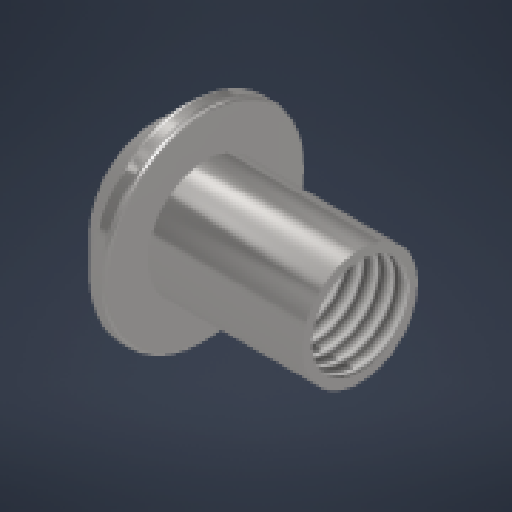
# Autodesk Inventor part: AliM5-8mm
Saved by Autodesk Inventor 2024.3 (Build 283343000, 343)
## iProperties
Created: 2024-06-23
Part Number: AliM5-8mm
Material: 스테인리스스틸
Catalog Web Link: www.cadenas.de
Description: DBB, DBM, DBS, DBSY-Stepped Screws - Low Head Selectable
Vendor: MISUMI
Document SubType Name: Modeling
Designer: ASUS
Manufacturer: MISUMI
Mass: 3.5682 g
Surface Area: 4.58831 cm^2
Volume: 0.446026 cm^3
Density: 8 g/cm^3
Appearance: 반연마
Category: PARTsolutions
Company: MISUMI
Title: DBSY4-5-8
Author: Cadenas PARTsolutions
Comments: Stepped Screws - Low Head Selectable
PSOL_IDENT_0: {$CADENAS_DATA/23d-libs/misumi/metric/27_screws_nuts/dbb.prj},184 {VTYP=3D},{NB=DBSY4-5-8},{LINA=DBS
PSOL_IDENT_1: Y4-5-8},{NN=DBB, DBM, DBS, DBSY},{DATE=29.05.2023 07:54:54},{GEOMDATE=17.01.2022 08:24:34},{VERSION=
PSOL_IDENT_2: },{LINEID=20},{WBVAR=MAT,ST,L,F},{WBNUMERIC=L,F}  {NB=DBSY4-5-8},{LINA=DBSY4-5-8},{KT=DUMMY},{PN=DBS
PSOL_IDENT_3: Y4-5-8},{TYPE=DB},{MAT=SY},{ST=-},{STALG= '-','-'},{M=4},{L=5},{LALG=3,4,5,6,7,8,10},{F=8},{FALG=4,5
PSOL_IDENT_4: ,6,8},{E=2.8},{DHH7=6},{A=10},{B=2.5},{LL=1.2},{HH1=2.5}
NB: DBSY4-5-8
NN: DBB, DBM, DBS, DBSY
NT: Stepped Screws - Low Head Selectable
NBSYN: $PN.
LINA: DBSY4-5-8
CATALOG: Misumi
PN: DBSY4-5-8
TYPE: DB
MAT: 304 Stainless Steel
ST: -
M: 4
L: 5
F: 8
E: 2.8
DHH7: 6
A: 10
B: 2.5
LL: 1.2
HH1: 2.5
SUPPLIER: MISUMI
ARTICLENO: DBSY4-5-8
BOMINFO: DBSY4-5-8
CREATOR: CADENAS GmbH
Autodesk Inventor part; units mm, degrees
ref_plane "YZ Plane" through (0, 0, 0) normal (1, 0, 0) x (0, 1, 0)
ref_plane "XZ Plane" through (0, 0, 0) normal (0, 1, 0) x (-1, 0, 0)
ref_plane "XY Plane" through (0, 0, 0) normal (0, 0, 1) x (1, 0, 0)
sketch "Sketch_1" plane through (0, 0, 0) normal (0, 0, 1) x (1, 0, 0)
  line L0 (8, 0) -> (-7.8, 0)
  line L1 (-7.8, 0) -> (-7.8, 5)
  line L2 (-7.8, 5) -> (-5, 5)
  line L3 (-5, 5) -> (-5, 3)
  line L4 (-5, 3) -> (0, 3)
  line L5 (0, 3) -> (0, 2)
  line L6 (0, 2) -> (7.5705, 2)
  line L7 (7.5705, 2) -> (8, 1.5705)
  line L8 (8, 1.5705) -> (8, 0)
  line L9 (8, 0) -> (-7.8, 0)
  constraints: 20 end point
revolve "Revolution1" add sketch "Sketch_1" angle 360 about axis through (8, 0, 0) along (1, 0, 0)
thread "Thread1" size "M4x0.7" class "6g" standard "ISO Metric profile" length 6.3705
sketch "Sketch_2" plane through (-7.8, 0, 0) normal (-1, 0, 0) x (0, 1, 0)
  line L0 (-1.4434, 0) -> (-0.7217, -1.25)
  line L1 (-0.7217, -1.25) -> (0.7217, -1.25)
  line L2 (0.7217, -1.25) -> (1.4434, 0)
  line L3 (1.4434, 0) -> (0.7217, 1.25)
  line L4 (0.7217, 1.25) -> (-0.7217, 1.25)
  line L5 (-0.7217, 1.25) -> (-1.4434, 0)
  constraints: 12 end point
extrude "Extrusion1" cut sketch "Sketch_2" against normal blind 2.5
sketch "Sketch_3" plane through (0, 0, 0) normal (0, 0, 1) x (1, 0, 0)
  line L0 (-4.5783, 0) -> (-5.3, 0)
  line L1 (-5.3, 0) -> (-5.3, 1.25)
  line L2 (-5.3, 1.25) -> (-4.5783, 0)
  line L3 (-4.5783, 0) -> (-5.3, 0)
  constraints: 8 end point
revolve "Revolution2" cut sketch "Sketch_3" angle 360 about axis through (-4.5783, 0, 0) along (1, 0, 0)
sketch "스케치4" plane through (0, 0, 0) normal (1, 0, 0) x (0, 0, -1)
  circle A0 centre (0, 0) radius 2 projected
  circle A1 centre (0, 0) radius 3 projected
extrude "돌출2" add sketch "스케치4" along normal blind 3 contours A0 | A1
sketch "스케치5" plane through (8, 0, 0) normal (1, 0, 0) x (0, 0, -1)
  circle A0 centre (0, 0) radius 1.5705 projected
  circle A1 centre (0, 0) radius 2.5
  dimension "d8" = 5
  constraints: 1 centre point, 1 coincident
  measures "d8" diameter of A1
extrude "돌출3" cut sketch "스케치5" against normal blind 11 contours A0 | A1
sketch "스케치6" plane through (-5, 0, 0) normal (1, 0, 0) x (0, 0, -1)
  circle A0 centre (0, 0) radius 3 projected
  circle A1 centre (0, 0) radius 5 projected
  circle A2 centre (0, 0) radius 5.25
  dimension "d11" = 10.5
  constraints: 1 centre point, 1 coincident
  measures "d11" diameter of A2
extrude "돌출4" add sketch "스케치6" against normal up to surface (2.8 mm away) contours A2
chamfer "모따기1" distance 2 angle 45 1 edges at (-7.8, 0, 5.25)
fillet "모깎기1" radius 0.25 3 edges at (-7.8, 0, 3.25) (-5.8, 0, 5.25) (-5, 0, 5.25)
thread "스레드2" size "M5x0.8" class "6H" standard "ANSI Metric M Profile" full length
body "Solid1"
